Autodesk Inventor part; units mm, degrees
(part 3 of 3)
  spline S71 degree 3 poles (611.9865, 25.0748) (610.6815, 25.5594) (608.0715, 26.5286) (604.1238, 27.8919) (600.1524, 29.1842) (596.1558, 30.3968) (592.133, 31.5183) (589.1016, 32.3079) (587.0663, 32.7741) (586.2405, 33.0576) (585.6183, 33.3719) (585.1825, 33.6602) (584.7659, 33.9763) (584.3992, 34.3495) (584.0638, 34.7502) (583.7778, 35.1888) (583.5529, 35.6608) (583.3681, 36.1496) (583.2424, 36.658) (583.1703, 37.3513) (583.1308, 38.2204) (583.0565, 39.0872) (583.0375, 39.784) (583.0958, 40.3045) (583.2151, 40.8133) (583.3766, 41.3106) (583.6029, 41.7827) (583.883, 42.2238) (584.1979, 42.6417) (584.5697, 43.0094) (584.9641, 43.3521) (585.54, 43.745) (586.3218, 44.1338) (588.2787, 44.8617) (591.1811, 46.0402) (595.0232, 47.6772) (598.8274, 49.4011) (602.596, 51.2007) (606.332, 53.0676) (608.7932, 54.3692) (610.0238, 55.02) knots 0 0 0 0 0.062504 0.125008 0.187512 0.250016 0.31252 0.375023 0.390648 0.406259 0.414073 0.421883 0.429693 0.437504 0.445316 0.453129 0.460938 0.468749 0.476563 0.484374 0.5 0.515626 0.523437 0.531251 0.539062 0.546871 0.554684 0.562496 0.570307 0.578117 0.585927 0.593741 0.609352 0.624977 0.68748 0.749984 0.812488 0.874992 0.937496 1 1 1 1 projected
  arc A75 (610.0238, 55.02) -> (609.0362, 65.0469) centre (0, 0) ccw projected
  spline S72 degree 3 poles (609.0362, 65.0469) (607.7023, 65.4451) (605.0345, 66.2416) (601.0061, 67.3437) (596.9587, 68.3736) (592.8914, 69.3221) (588.8038, 70.1781) (585.7272, 70.7678) (583.6659, 71.0999) (582.8232, 71.3287) (582.1818, 71.6018) (581.7281, 71.8609) (581.2917, 72.1491) (580.9014, 72.4975) (580.5405, 72.8754) (580.2265, 73.2943) (579.9711, 73.7506) (579.7548, 74.2263) (579.5961, 74.7254) (579.4788, 75.4125) (579.3825, 76.2772) (579.2517, 77.1372) (579.1872, 77.8313) (579.2113, 78.3545) (579.2971, 78.87) (579.4257, 79.3768) (579.6206, 79.8627) (579.8713, 80.3212) (580.1582, 80.7587) (580.5051, 81.15) (580.8763, 81.5177) (581.4252, 81.9475) (582.1799, 82.3866) (584.0851, 83.2409) (586.9042, 84.6067) (590.631, 86.4915) (594.3142, 88.4605) (597.9571, 90.5028) (601.5631, 92.61) (603.9338, 94.0698) (605.1192, 94.7997) knots 0 0 0 0 0.062504 0.125008 0.187512 0.250016 0.31252 0.375023 0.390648 0.406259 0.414073 0.421883 0.429693 0.437504 0.445316 0.453129 0.460938 0.468749 0.476563 0.484374 0.5 0.515626 0.523437 0.531251 0.539062 0.546871 0.554684 0.562496 0.570307 0.578117 0.585927 0.593741 0.609352 0.624977 0.68748 0.749984 0.812488 0.874992 0.937496 1 1 1 1 projected
  arc A76 (605.1192, 94.7997) -> (603.478, 104.7405) centre (0, 0) ccw projected
  spline S73 degree 3 poles (603.478, 104.7405) (602.1209, 105.0506) (599.4067, 105.6709) (595.3148, 106.5072) (591.2087, 107.2701) (587.088, 107.9507) (582.9532, 108.5375) (579.8447, 108.9247) (577.766, 109.1212) (576.9102, 109.2945) (576.2523, 109.525) (575.7826, 109.7539) (575.3283, 110.0129) (574.916, 110.335) (574.5313, 110.6885) (574.1905, 111.086) (573.9058, 111.5246) (573.6589, 111.9851) (573.4678, 112.4728) (573.3059, 113.1508) (573.1532, 114.0073) (572.9665, 114.857) (572.8567, 115.5453) (572.8465, 116.069) (572.8985, 116.5889) (572.9936, 117.1031) (573.1564, 117.6007) (573.3765, 118.0746) (573.6342, 118.53) (573.9548, 118.9431) (574.3011, 119.3343) (574.8207, 119.7991) (575.5451, 120.2866) (577.3903, 121.2637) (580.114, 122.811) (583.7096, 124.9355) (587.2562, 127.1411) (590.7577, 129.4173) (594.2181, 131.7558) (596.4883, 133.3675) (597.6234, 134.1734) knots 0 0 0 0 0.062504 0.125008 0.187512 0.250016 0.31252 0.375023 0.390648 0.406259 0.414073 0.421883 0.429693 0.437504 0.445316 0.453129 0.460938 0.468749 0.476563 0.484374 0.5 0.515626 0.523437 0.531251 0.539062 0.546871 0.554684 0.562496 0.570307 0.578117 0.585927 0.593741 0.609352 0.624977 0.68748 0.749984 0.812488 0.874992 0.937496 1 1 1 1 projected
  arc A77 (597.6234, 134.1734) -> (595.3355, 143.9856) centre (0, 0) ccw projected
  spline S74 degree 3 poles (595.3355, 143.9856) (593.9611, 144.2063) (591.2121, 144.6477) (587.0743, 145.2146) (582.9271, 145.7074) (578.7707, 146.1169) (574.6064, 146.4321) (571.4792, 146.6151) (569.3921, 146.6753) (568.5268, 146.7922) (567.8552, 146.9792) (567.3716, 147.1769) (566.9013, 147.4056) (566.4688, 147.7001) (566.0618, 148.0277) (565.6957, 148.402) (565.383, 148.8211) (565.1064, 149.2645) (564.8839, 149.7386) (564.6779, 150.4045) (564.4696, 151.2492) (564.2277, 152.0848) (564.0731, 152.7645) (564.0288, 153.2864) (564.0466, 153.8087) (564.1079, 154.3279) (564.2377, 154.8352) (564.4264, 155.3224) (564.6538, 155.7937) (564.9466, 156.2269) (565.2666, 156.6399) (565.7548, 157.1376) (566.4457, 157.6715) (568.223, 158.7672) (570.8398, 160.4893) (574.2886, 162.8444) (577.6834, 165.2773) (581.0285, 167.7776) (584.3286, 170.3374) (586.4885, 172.0942) (587.5685, 172.9726) knots 0 0 0 0 0.062504 0.125008 0.187512 0.250016 0.31252 0.375023 0.390648 0.406259 0.414073 0.421883 0.429693 0.437504 0.445316 0.453129 0.460938 0.468749 0.476563 0.484374 0.5 0.515626 0.523437 0.531251 0.539062 0.546871 0.554684 0.562496 0.570307 0.578117 0.585927 0.593741 0.609352 0.624977 0.68748 0.749984 0.812488 0.874992 0.937496 1 1 1 1 projected
  arc A78 (587.5685, 172.9726) -> (584.6438, 182.6141) centre (0, 0) ccw projected
  spline S75 degree 3 poles (584.6438, 182.6141) (583.2578, 182.7445) (580.4859, 183.0051) (576.3198, 183.3002) (572.1493, 183.5207) (567.975, 183.6575) (563.799, 183.6996) (560.6665, 183.6777) (558.58, 183.6013) (557.7089, 183.6613) (557.0265, 183.804) (556.531, 183.9696) (556.0468, 184.1671) (555.5959, 184.4327) (555.1683, 184.733) (554.7786, 185.0826) (554.4391, 185.4802) (554.1341, 185.9046) (553.8811, 186.3632) (553.632, 187.0142) (553.3689, 187.8434) (553.0728, 188.6615) (552.8741, 189.3296) (552.7957, 189.8475) (552.7793, 190.3698) (552.8066, 190.8919) (552.903, 191.4066) (553.0594, 191.9051) (553.2554, 192.3902) (553.5193, 192.8417) (553.8116, 193.2747) (554.2662, 193.8033) (554.9207, 194.3813) (556.6226, 195.5908) (559.121, 197.4804) (562.4085, 200.056) (565.6369, 202.7057) (568.8113, 205.4194) (571.9369, 208.1897) (573.9773, 210.0839) (574.9975, 211.031) knots 0 0 0 0 0.062504 0.125008 0.187512 0.250016 0.31252 0.375023 0.390648 0.406259 0.414073 0.421883 0.429693 0.437504 0.445316 0.453129 0.460938 0.468749 0.476563 0.484374 0.5 0.515626 0.523437 0.531251 0.539062 0.546871 0.554684 0.562496 0.570307 0.578117 0.585927 0.593741 0.609352 0.624977 0.68748 0.749984 0.812488 0.874992 0.937496 1 1 1 1 projected
  arc A79 (574.9975, 211.031) -> (571.4485, 220.4607) centre (0, 0) ccw projected
  spline S76 degree 3 poles (571.4485, 220.4607) (570.0569, 220.5001) (567.2739, 220.5789) (563.0974, 220.6009) (558.9215, 220.5481) (554.7472, 220.4116) (550.5773, 220.1805) (547.453, 219.9538) (545.3759, 219.741) (544.5028, 219.744) (543.8125, 219.8417) (543.3072, 219.9746) (542.8111, 220.14) (542.3439, 220.3755) (541.8976, 220.6472) (541.4858, 220.9705) (541.121, 221.3452) (540.7889, 221.7487) (540.5064, 222.1897) (540.2153, 222.823) (539.8985, 223.6333) (539.5496, 224.4302) (539.3076, 225.0839) (539.1955, 225.5955) (539.145, 226.1157) (539.138, 226.6385) (539.2006, 227.1583) (539.3241, 227.666) (539.4879, 228.1629) (539.7217, 228.6307) (539.9851, 229.0819) (540.4041, 229.6391) (541.0194, 230.2586) (542.6385, 231.5769) (545.0081, 233.6258) (548.12, 236.411) (551.1682, 239.2661) (554.1584, 242.1816) (557.0961, 245.1504) (559.0082, 247.174) (559.9643, 248.1858) knots 0 0 0 0 0.062504 0.125008 0.187512 0.250016 0.31252 0.375023 0.390648 0.406259 0.414073 0.421883 0.429693 0.437504 0.445316 0.453129 0.460938 0.468749 0.476563 0.484374 0.5 0.515626 0.523437 0.531251 0.539062 0.546871 0.554684 0.562496 0.570307 0.578117 0.585927 0.593741 0.609352 0.624977 0.68748 0.749984 0.812488 0.874992 0.937496 1 1 1 1 projected
  arc A80 (559.9643, 248.1858) -> (555.8061, 257.3632) centre (0, 0) ccw projected
  spline S77 degree 3 poles (555.8061, 257.3632) (554.415, 257.3115) (551.6328, 257.2081) (547.4638, 256.9569) (543.3002, 256.6311) (539.1438, 256.2219) (534.998, 255.7186) (531.8952, 255.288) (529.8365, 254.9399) (528.965, 254.8857) (528.2698, 254.9381) (527.7569, 255.0376) (527.2511, 255.1702) (526.7694, 255.3746) (526.3063, 255.6166) (525.8742, 255.9123) (525.4858, 256.2623) (525.128, 256.6432) (524.8173, 257.0648) (524.4854, 257.6777) (524.1162, 258.4655) (523.7159, 259.2379) (523.4317, 259.8744) (523.2864, 260.3776) (523.202, 260.8933) (523.1608, 261.4146) (523.1892, 261.9374) (523.2793, 262.4521) (523.4103, 262.9586) (523.613, 263.4407) (523.8463, 263.9082) (524.2279, 264.4916) (524.8014, 265.15) (526.3309, 266.5713) (528.5613, 268.7708) (531.4845, 271.7535) (534.3394, 274.802) (537.1325, 277.9068) (539.8697, 281.0613) (541.6454, 283.2057) (542.5333, 284.2779) knots 0 0 0 0 0.062504 0.125008 0.187512 0.250016 0.31252 0.375023 0.390648 0.406259 0.414073 0.421883 0.429693 0.437504 0.445316 0.453129 0.460938 0.468749 0.476563 0.484374 0.5 0.515626 0.523437 0.531251 0.539062 0.546871 0.554684 0.562496 0.570307 0.578117 0.585927 0.593741 0.609352 0.624977 0.68748 0.749984 0.812488 0.874992 0.937496 1 1 1 1 projected
  arc A81 (542.5333, 284.2779) -> (537.7837, 293.1636) centre (0, 0) ccw projected
  spline S78 degree 3 poles (537.7837, 293.1636) (536.399, 293.021) (533.6295, 292.7359) (529.4859, 292.2126) (525.3525, 291.6152) (521.2318, 290.935) (517.1277, 290.1616) (514.0597, 289.529) (512.0282, 289.047) (511.1621, 288.936) (510.465, 288.9427) (509.9467, 289.0085) (509.4333, 289.1077) (508.9393, 289.2802) (508.4613, 289.4913) (508.0108, 289.7582) (507.6003, 290.082) (507.2184, 290.4387) (506.8808, 290.8391) (506.5095, 291.429) (506.0896, 292.191) (505.6397, 292.9356) (505.3144, 293.5521) (505.1365, 294.0447) (505.0185, 294.5538) (504.9434, 295.0712) (504.9375, 295.5947) (504.9937, 296.1142) (505.0913, 296.6283) (505.2621, 297.1225) (505.4643, 297.6043) (505.8069, 298.2114) (506.3361, 298.9059) (507.7693, 300.4243) (509.8512, 302.765) (512.573, 305.9324) (515.2224, 309.161) (517.8064, 312.4419) (520.3315, 315.7687) (521.9632, 318.0246) (522.779, 319.1526) knots 0 0 0 0 0.062504 0.125008 0.187512 0.250016 0.31252 0.375023 0.390648 0.406259 0.414073 0.421883 0.429693 0.437504 0.445316 0.453129 0.460938 0.468749 0.476563 0.484374 0.5 0.515626 0.523437 0.531251 0.539062 0.546871 0.554684 0.562496 0.570307 0.578117 0.585927 0.593741 0.609352 0.624977 0.68748 0.749984 0.812488 0.874992 0.937496 1 1 1 1 projected
  arc A82 (522.779, 319.1526) -> (517.4585, 327.7086) centre (0, 0) ccw projected
  spline S79 degree 3 poles (517.4585, 327.7086) (516.086, 327.4758) (513.3411, 327.0102) (509.2406, 326.217) (505.1551, 325.3505) (501.0877, 324.4023) (497.043, 323.3621) (494.023, 322.5302) (492.0273, 321.9163) (491.1704, 321.7489) (490.4743, 321.7101) (489.9528, 321.7418) (489.434, 321.8073) (488.9298, 321.9471) (488.439, 322.1265) (487.9721, 322.3633) (487.5412, 322.6596) (487.1368, 322.9905) (486.7737, 323.368) (486.3646, 323.9323) (485.8958, 324.6652) (485.3981, 325.3788) (485.0333, 325.9727) (484.8235, 326.4526) (484.6725, 326.9529) (484.5637, 327.4643) (484.5236, 327.9863) (484.5457, 328.5084) (484.6094, 329.0277) (484.7475, 329.5321) (484.9178, 330.0261) (485.22, 330.6543) (485.7026, 331.3819) (487.0335, 332.9907) (488.9578, 335.4626) (491.4666, 338.8013) (493.8992, 342.1963) (496.2631, 345.6391) (498.5651, 349.1239) (500.0458, 351.4817) (500.7861, 352.6606) knots 0 0 0 0 0.062504 0.125008 0.187512 0.250016 0.31252 0.375023 0.390648 0.406259 0.414073 0.421883 0.429693 0.437504 0.445316 0.453129 0.460938 0.468749 0.476563 0.484374 0.5 0.515626 0.523437 0.531251 0.539062 0.546871 0.554684 0.562496 0.570307 0.578117 0.585927 0.593741 0.609352 0.624977 0.68748 0.749984 0.812488 0.874992 0.937496 1 1 1 1 projected
  arc A83 (500.7861, 352.6606) -> (494.9174, 360.8504) centre (0, 0) ccw projected
  spline S80 degree 3 poles (494.9174, 360.8504) (493.5631, 360.5283) (490.8545, 359.8842) (486.8147, 358.8244) (482.7946, 357.6926) (478.7979, 356.4804) (474.8299, 355.1779) (471.8707, 354.1503) (469.9195, 353.4072) (469.0753, 353.1841) (468.3833, 353.0998) (467.8609, 353.0974) (467.3389, 353.1288) (466.8266, 353.2353) (466.3252, 353.3822) (465.8437, 353.588) (465.3944, 353.8554) (464.9692, 354.1592) (464.5822, 354.5121) (464.1371, 355.0485) (463.6214, 355.7492) (463.0781, 356.4287) (462.6752, 356.9975) (462.4345, 357.4626) (462.251, 357.952) (462.109, 358.4552) (462.0348, 358.9735) (462.0227, 359.4958) (462.0524, 360.0182) (462.1572, 360.5306) (462.2948, 361.0346) (462.5553, 361.6812) (462.9893, 362.4389) (464.2121, 364.1313) (465.9706, 366.7237) (468.2556, 370.2193) (470.461, 373.7661) (472.5947, 377.3563) (474.6639, 380.9841) (475.9871, 383.4337) (476.6488, 384.6585) knots 0 0 0 0 0.062504 0.125008 0.187512 0.250016 0.31252 0.375023 0.390648 0.406259 0.414073 0.421883 0.429693 0.437504 0.445316 0.453129 0.460938 0.468749 0.476563 0.484374 0.5 0.515626 0.523437 0.531251 0.539062 0.546871 0.554684 0.562496 0.570307 0.578117 0.585927 0.593741 0.609352 0.624977 0.68748 0.749984 0.812488 0.874992 0.937496 1 1 1 1 projected
  arc A84 (476.6488, 384.6585) -> (470.257, 392.4469) centre (0, 0) ccw projected
  spline S81 degree 3 poles (470.257, 392.4469) (468.9267, 392.037) (466.266, 391.217) (462.3041, 389.8954) (458.3667, 388.503) (454.4578, 387.032) (450.5835, 385.4728) (447.6979, 384.2539) (445.7994, 383.3848) (444.9717, 383.1069) (444.2867, 382.9776) (443.7655, 382.941) (443.2425, 382.9381) (442.7244, 383.0109) (442.2144, 383.1247) (441.7205, 383.2986) (441.2547, 383.5361) (440.8106, 383.8114) (440.4013, 384.1382) (439.922, 384.6444) (439.3616, 385.3098) (438.775, 385.9523) (438.3358, 386.4935) (438.0652, 386.9419) (437.8501, 387.4182) (437.6755, 387.9111) (437.5676, 388.4234) (437.5214, 388.9439) (437.5168, 389.4671) (437.5879, 389.9852) (437.6922, 390.4971) (437.9098, 391.1594) (438.2934, 391.9438) (439.4028, 393.7126) (440.988, 396.4144) (443.0396, 400.0521) (445.0082, 403.7355) (446.9025, 407.4575) (448.73, 411.2129) (449.8903, 413.7438) (450.4704, 415.0093) knots 0 0 0 0 0.062504 0.125008 0.187512 0.250016 0.31252 0.375023 0.390648 0.406259 0.414073 0.421883 0.429693 0.437504 0.445316 0.453129 0.460938 0.468749 0.476563 0.484374 0.5 0.515626 0.523437 0.531251 0.539062 0.546871 0.554684 0.562496 0.570307 0.578117 0.585927 0.593741 0.609352 0.624977 0.68748 0.749984 0.812488 0.874992 0.937496 1 1 1 1 projected
  arc A85 (450.4704, 415.0093) -> (443.5829, 422.363) centre (0, 0) ccw projected
  spline S82 degree 3 poles (443.5829, 422.363) (442.2822, 421.8669) (439.6808, 420.8747) (435.8139, 419.2967) (431.976, 417.6498) (428.1717, 415.9263) (424.4077, 414.1171) (421.6079, 412.712) (419.7704, 411.7206) (418.9626, 411.3892) (418.2875, 411.2153) (417.7698, 411.1447) (417.2482, 411.1077) (416.7264, 411.1464) (416.21, 411.2266) (415.7059, 411.3678) (415.2255, 411.5743) (414.7643, 411.82) (414.3345, 412.1194) (413.8232, 412.5931) (413.2204, 413.2204) (412.5931, 413.8232) (412.1194, 414.3345) (411.82, 414.7643) (411.5743, 415.2255) (411.3678, 415.7059) (411.2266, 416.21) (411.1464, 416.7264) (411.1077, 417.2482) (411.1447, 417.7698) (411.2153, 418.2875) (411.3892, 418.9626) (411.7206, 419.7704) (412.712, 421.6079) (414.1171, 424.4077) (415.9263, 428.1717) (417.6498, 431.976) (419.2967, 435.8139) (420.8747, 439.6808) (421.8669, 442.2822) (422.363, 443.5829) knots 0 0 0 0 0.062504 0.125008 0.187512 0.250016 0.31252 0.375023 0.390648 0.406259 0.414073 0.421883 0.429693 0.437504 0.445316 0.453129 0.460938 0.468749 0.476563 0.484374 0.5 0.515626 0.523437 0.531251 0.539062 0.546871 0.554684 0.562496 0.570307 0.578117 0.585927 0.593741 0.609352 0.624977 0.68748 0.749984 0.812488 0.874992 0.937496 1 1 1 1 projected
  arc A86 (422.363, 443.5829) -> (415.0093, 450.4704) centre (0, 0) ccw projected
  spline S83 degree 3 poles (415.0093, 450.4704) (413.7438, 449.8903) (411.2129, 448.73) (407.4575, 446.9025) (403.7355, 445.0082) (400.0521, 443.0396) (396.4144, 440.988) (393.7126, 439.4028) (391.9438, 438.2934) (391.1594, 437.9098) (390.4971, 437.6922) (389.9852, 437.5879) (389.4671, 437.5168) (388.9439, 437.5214) (388.4234, 437.5676) (387.9111, 437.6755) (387.4182, 437.8501) (386.9419, 438.0652) (386.4935, 438.3358) (385.9523, 438.775) (385.3098, 439.3616) (384.6444, 439.922) (384.1382, 440.4013) (383.8114, 440.8106) (383.5361, 441.2547) (383.2986, 441.7205) (383.1247, 442.2144) (383.0109, 442.7244) (382.9381, 443.2425) (382.941, 443.7655) (382.9776, 444.2867) (383.1069, 444.9717) (383.3848, 445.7994) (384.2539, 447.6979) (385.4728, 450.5835) (387.032, 454.4578) (388.503, 458.3667) (389.8954, 462.3041) (391.217, 466.266) (392.037, 468.9267) (392.4469, 470.257) knots 0 0 0 0 0.062504 0.125008 0.187512 0.250016 0.31252 0.375023 0.390648 0.406259 0.414073 0.421883 0.429693 0.437504 0.445316 0.453129 0.460938 0.468749 0.476563 0.484374 0.5 0.515626 0.523437 0.531251 0.539062 0.546871 0.554684 0.562496 0.570307 0.578117 0.585927 0.593741 0.609352 0.624977 0.68748 0.749984 0.812488 0.874992 0.937496 1 1 1 1 projected
  arc A87 (392.4469, 470.257) -> (384.6585, 476.6488) centre (0, 0) ccw projected
  spline S84 degree 3 poles (384.6585, 476.6488) (383.4337, 475.9871) (380.9841, 474.6639) (377.3563, 472.5947) (373.7661, 470.461) (370.2193, 468.2556) (366.7237, 465.9706) (364.1313, 464.2121) (362.4389, 462.9893) (361.6812, 462.5553) (361.0346, 462.2948) (360.5306, 462.1572) (360.0182, 462.0524) (359.4958, 462.0227) (358.9735, 462.0348) (358.4552, 462.109) (357.952, 462.251) (357.4626, 462.4345) (356.9975, 462.6752) (356.4287, 463.0781) (355.7492, 463.6214) (355.0485, 464.1371) (354.5121, 464.5822) (354.1592, 464.9692) (353.8554, 465.3944) (353.588, 465.8437) (353.3822, 466.3252) (353.2353, 466.8266) (353.1288, 467.3389) (353.0974, 467.8609) (353.0998, 468.3833) (353.1841, 469.0753) (353.4072, 469.9195) (354.1503, 471.8707) (355.1779, 474.8299) (356.4804, 478.7979) (357.6926, 482.7946) (358.8244, 486.8147) (359.8842, 490.8545) (360.5283, 493.5631) (360.8504, 494.9174) knots 0 0 0 0 0.062504 0.125008 0.187512 0.250016 0.31252 0.375023 0.390648 0.406259 0.414073 0.421883 0.429693 0.437504 0.445316 0.453129 0.460938 0.468749 0.476563 0.484374 0.5 0.515626 0.523437 0.531251 0.539062 0.546871 0.554684 0.562496 0.570307 0.578117 0.585927 0.593741 0.609352 0.624977 0.68748 0.749984 0.812488 0.874992 0.937496 1 1 1 1 projected
  arc A88 (360.8504, 494.9174) -> (352.6606, 500.7861) centre (0, 0) ccw projected
  spline S85 degree 3 poles (352.6606, 500.7861) (351.4817, 500.0458) (349.1239, 498.5651) (345.6391, 496.2631) (342.1963, 493.8992) (338.8013, 491.4666) (335.4626, 488.9578) (332.9907, 487.0335) (331.3819, 485.7026) (330.6543, 485.22) (330.0261, 484.9178) (329.5321, 484.7475) (329.0277, 484.6094) (328.5084, 484.5457) (327.9863, 484.5236) (327.4643, 484.5637) (326.9529, 484.6725) (326.4526, 484.8235) (325.9727, 485.0333) (325.3788, 485.3981) (324.6652, 485.8958) (323.9323, 486.3646) (323.368, 486.7737) (322.9905, 487.1368) (322.6596, 487.5412) (322.3633, 487.9721) (322.1265, 488.439) (321.9471, 488.9298) (321.8073, 489.434) (321.7418, 489.9528) (321.7101, 490.4743) (321.7489, 491.1704) (321.9163, 492.0273) (322.5302, 494.023) (323.3621, 497.043) (324.4023, 501.0877) (325.3505, 505.1551) (326.217, 509.2406) (327.0102, 513.3411) (327.4758, 516.086) (327.7086, 517.4585) knots 0 0 0 0 0.062504 0.125008 0.187512 0.250016 0.31252 0.375023 0.390648 0.406259 0.414073 0.421883 0.429693 0.437504 0.445316 0.453129 0.460938 0.468749 0.476563 0.484374 0.5 0.515626 0.523437 0.531251 0.539062 0.546871 0.554684 0.562496 0.570307 0.578117 0.585927 0.593741 0.609352 0.624977 0.68748 0.749984 0.812488 0.874992 0.937496 1 1 1 1 projected
  arc A89 (327.7086, 517.4585) -> (319.1526, 522.779) centre (0, 0) ccw projected
  spline S86 degree 3 poles (319.1526, 522.779) (318.0246, 521.9632) (315.7687, 520.3315) (312.4419, 517.8064) (309.161, 515.2224) (305.9324, 512.573) (302.765, 509.8512) (300.4243, 507.7693) (298.9059, 506.3361) (298.2114, 505.8069) (297.6043, 505.4643) (297.1225, 505.2621) (296.6283, 505.0913) (296.1142, 504.9937) (295.5947, 504.9375) (295.0712, 504.9434) (294.5538, 505.0185) (294.0447, 505.1365) (293.5521, 505.3144) (292.9356, 505.6397) (292.191, 506.0896) (291.429, 506.5095) (290.8391, 506.8808) (290.4387, 507.2184) (290.082, 507.6003) (289.7582, 508.0108) (289.4913, 508.4613) (289.2802, 508.9393) (289.1077, 509.4333) (289.0085, 509.9467) (288.9427, 510.465) (288.936, 511.1621) (289.047, 512.0282) (289.529, 514.0597) (290.1616, 517.1277) (290.935, 521.2318) (291.6152, 525.3525) (292.2126, 529.4859) (292.7359, 533.6295) (293.021, 536.399) (293.1636, 537.7837) knots 0 0 0 0 0.062504 0.125008 0.187512 0.250016 0.31252 0.375023 0.390648 0.406259 0.414073 0.421883 0.429693 0.437504 0.445316 0.453129 0.460938 0.468749 0.476563 0.484374 0.5 0.515626 0.523437 0.531251 0.539062 0.546871 0.554684 0.562496 0.570307 0.578117 0.585927 0.593741 0.609352 0.624977 0.68748 0.749984 0.812488 0.874992 0.937496 1 1 1 1 projected
  arc A90 (293.1636, 537.7837) -> (284.2779, 542.5333) centre (0, 0) ccw projected
  spline S87 degree 3 poles (284.2779, 542.5333) (283.2057, 541.6454) (281.0613, 539.8697) (277.9068, 537.1325) (274.802, 534.3394) (271.7535, 531.4845) (268.7708, 528.5613) (266.5713, 526.3309) (265.15, 524.8014) (264.4916, 524.2279) (263.9082, 523.8463) (263.4407, 523.613) (262.9586, 523.4103) (262.4521, 523.2793) (261.9374, 523.1892) (261.4146, 523.1608) (260.8933, 523.202) (260.3776, 523.2864) (259.8744, 523.4317) (259.2379, 523.7159) (258.4655, 524.1162) (257.6777, 524.4854) (257.0648, 524.8173) (256.6432, 525.128) (256.2623, 525.4858) (255.9123, 525.8742) (255.6166, 526.3063) (255.3746, 526.7694) (255.1702, 527.2511) (255.0376, 527.7569) (254.9381, 528.2698) (254.8857, 528.965) (254.9399, 529.8365) (255.288, 531.8952) (255.7186, 534.998) (256.2219, 539.1438) (256.6311, 543.3002) (256.9569, 547.4638) (257.2081, 551.6328) (257.3115, 554.415) (257.3632, 555.8061) knots 0 0 0 0 0.062504 0.125008 0.187512 0.250016 0.31252 0.375023 0.390648 0.406259 0.414073 0.421883 0.429693 0.437504 0.445316 0.453129 0.460938 0.468749 0.476563 0.484374 0.5 0.515626 0.523437 0.531251 0.539062 0.546871 0.554684 0.562496 0.570307 0.578117 0.585927 0.593741 0.609352 0.624977 0.68748 0.749984 0.812488 0.874992 0.937496 1 1 1 1 projected
  arc A91 (257.3632, 555.8061) -> (248.1858, 559.9643) centre (0, 0) ccw projected
  spline S88 degree 3 poles (248.1858, 559.9643) (247.174, 559.0082) (245.1504, 557.0961) (242.1816, 554.1584) (239.2661, 551.1682) (236.411, 548.12) (233.6258, 545.0081) (231.5769, 542.6385) (230.2586, 541.0194) (229.6391, 540.4041) (229.0819, 539.9851) (228.6307, 539.7217) (228.1629, 539.4879) (227.666, 539.3241) (227.1583, 539.2006) (226.6385, 539.138) (226.1157, 539.145) (225.5955, 539.1955) (225.0839, 539.3076) (224.4302, 539.5496) (223.6333, 539.8985) (222.823, 540.2153) (222.1897, 540.5064) (221.7487, 540.7889) (221.3452, 541.121) (220.9705, 541.4858) (220.6472, 541.8976) (220.3755, 542.3439) (220.14, 542.8111) (219.9746, 543.3072) (219.8417, 543.8125) (219.744, 544.5028) (219.741, 545.3759) (219.9538, 547.453) (220.1805, 550.5773) (220.4116, 554.7472) (220.5481, 558.9215) (220.6009, 563.0974) (220.5789, 567.2739) (220.5001, 570.0569) (220.4607, 571.4485) knots 0 0 0 0 0.062504 0.125008 0.187512 0.250016 0.31252 0.375023 0.390648 0.406259 0.414073 0.421883 0.429693 0.437504 0.445316 0.453129 0.460938 0.468749 0.476563 0.484374 0.5 0.515626 0.523437 0.531251 0.539062 0.546871 0.554684 0.562496 0.570307 0.578117 0.585927 0.593741 0.609352 0.624977 0.68748 0.749984 0.812488 0.874992 0.937496 1 1 1 1 projected
  arc A92 (220.4607, 571.4485) -> (211.031, 574.9975) centre (0, 0) ccw projected
  spline S89 degree 3 poles (211.031, 574.9975) (210.0839, 573.9773) (208.1897, 571.9369) (205.4194, 568.8113) (202.7057, 565.6369) (200.056, 562.4085) (197.4804, 559.121) (195.5908, 556.6226) (194.3813, 554.9207) (193.8033, 554.2662) (193.2747, 553.8116) (192.8417, 553.5193) (192.3902, 553.2554) (191.9051, 553.0594) (191.4066, 552.903) (190.8919, 552.8066) (190.3698, 552.7793) (189.8475, 552.7957) (189.3296, 552.8741) (188.6615, 553.0728) (187.8434, 553.3689) (187.0142, 553.632) (186.3632, 553.8811) (185.9046, 554.1341) (185.4802, 554.4391) (185.0826, 554.7786) (184.733, 555.1683) (184.4327, 555.5959) (184.1671, 556.0468) (183.9696, 556.531) (183.804, 557.0265) (183.6613, 557.7089) (183.6013, 558.58) (183.6777, 560.6665) (183.6996, 563.799) (183.6575, 567.975) (183.5207, 572.1493) (183.3002, 576.3198) (183.0051, 580.4859) (182.7445, 583.2578) (182.6141, 584.6438) knots 0 0 0 0 0.062504 0.125008 0.187512 0.250016 0.31252 0.375023 0.390648 0.406259 0.414073 0.421883 0.429693 0.437504 0.445316 0.453129 0.460938 0.468749 0.476563 0.484374 0.5 0.515626 0.523437 0.531251 0.539062 0.546871 0.554684 0.562496 0.570307 0.578117 0.585927 0.593741 0.609352 0.624977 0.68748 0.749984 0.812488 0.874992 0.937496 1 1 1 1 projected
  arc A93 (182.6141, 584.6438) -> (172.9726, 587.5685) centre (0, 0) ccw projected
  spline S90 degree 3 poles (172.9726, 587.5685) (172.0942, 586.4885) (170.3374, 584.3286) (167.7776, 581.0285) (165.2773, 577.6834) (162.8444, 574.2886) (160.4893, 570.8398) (158.7672, 568.223) (157.6715, 566.4457) (157.1376, 565.7548) (156.6399, 565.2666) (156.2269, 564.9466) (155.7937, 564.6538) (155.3224, 564.4264) (154.8352, 564.2377) (154.3279, 564.1079) (153.8087, 564.0466) (153.2864, 564.0288) (152.7645, 564.0731) (152.0848, 564.2277) (151.2492, 564.4696) (150.4045, 564.6779) (149.7386, 564.8839) (149.2645, 565.1064) (148.8211, 565.383) (148.402, 565.6957) (148.0277, 566.0618) (147.7001, 566.4688) (147.4056, 566.9013) (147.1769, 567.3716) (146.9792, 567.8552) (146.7922, 568.5268) (146.6753, 569.3921) (146.6151, 571.4792) (146.4321, 574.6064) (146.1169, 578.7707) (145.7074, 582.9271) (145.2146, 587.0743) (144.6477, 591.2121) (144.2063, 593.9611) (143.9856, 595.3355) knots 0 0 0 0 0.062504 0.125008 0.187512 0.250016 0.31252 0.375023 0.390648 0.406259 0.414073 0.421883 0.429693 0.437504 0.445316 0.453129 0.460938 0.468749 0.476563 0.484374 0.5 0.515626 0.523437 0.531251 0.539062 0.546871 0.554684 0.562496 0.570307 0.578117 0.585927 0.593741 0.609352 0.624977 0.68748 0.749984 0.812488 0.874992 0.937496 1 1 1 1 projected
  arc A94 (143.9856, 595.3355) -> (134.1734, 597.6234) centre (0, 0) ccw projected
  spline S91 degree 3 poles (134.1734, 597.6234) (133.3675, 596.4883) (131.7558, 594.2181) (129.4173, 590.7577) (127.1411, 587.2562) (124.9355, 583.7096) (122.811, 580.114) (121.2637, 577.3903) (120.2866, 575.5451) (119.7991, 574.8207) (119.3343, 574.3011) (118.9431, 573.9548) (118.53, 573.6342) (118.0746, 573.3765) (117.6007, 573.1564) (117.1031, 572.9936) (116.5889, 572.8985) (116.069, 572.8465) (115.5453, 572.8567) (114.857, 572.9665) (114.0073, 573.1532) (113.1508, 573.3059) (112.4728, 573.4678) (111.9851, 573.6589) (111.5246, 573.9058) (111.086, 574.1905) (110.6885, 574.5313) (110.335, 574.916) (110.0129, 575.3283) (109.7539, 575.7826) (109.525, 576.2523) (109.2945, 576.9102) (109.1212, 577.766) (108.9247, 579.8447) (108.5375, 582.9532) (107.9507, 587.088) (107.2701, 591.2087) (106.5072, 595.3148) (105.6709, 599.4067) (105.0506, 602.1209) (104.7405, 603.478) knots 0 0 0 0 0.062504 0.125008 0.187512 0.250016 0.31252 0.375023 0.390648 0.406259 0.414073 0.421883 0.429693 0.437504 0.445316 0.453129 0.460938 0.468749 0.476563 0.484374 0.5 0.515626 0.523437 0.531251 0.539062 0.546871 0.554684 0.562496 0.570307 0.578117 0.585927 0.593741 0.609352 0.624977 0.68748 0.749984 0.812488 0.874992 0.937496 1 1 1 1 projected
  arc A95 (104.7405, 603.478) -> (94.7997, 605.1192) centre (0, 0) ccw projected
  spline S92 degree 3 poles (94.7997, 605.1192) (94.0698, 603.9338) (92.61, 601.5631) (90.5028, 597.9571) (88.4605, 594.3142) (86.4915, 590.631) (84.6067, 586.9042) (83.2409, 584.0851) (82.3866, 582.1799) (81.9475, 581.4252) (81.5177, 580.8763) (81.15, 580.5051) (80.7587, 580.1582) (80.3212, 579.8713) (79.8627, 579.6206) (79.3768, 579.4257) (78.87, 579.2971) (78.3545, 579.2113) (77.8313, 579.1872) (77.1372, 579.2517) (76.2772, 579.3825) (75.4125, 579.4788) (74.7254, 579.5961) (74.2263, 579.7548) (73.7506, 579.9711) (73.2943, 580.2265) (72.8754, 580.5405) (72.4975, 580.9014) (72.1491, 581.2917) (71.8609, 581.7281) (71.6018, 582.1818) (71.3287, 582.8232) (71.0999, 583.6659) (70.7678, 585.7272) (70.1781, 588.8038) (69.3221, 592.8914) (68.3736, 596.9587) (67.3437, 601.0061) (66.2416, 605.0345) (65.4451, 607.7023) (65.0469, 609.0362) knots 0 0 0 0 0.062504 0.125008 0.187512 0.250016 0.31252 0.375023 0.390648 0.406259 0.414073 0.421883 0.429693 0.437504 0.445316 0.453129 0.460938 0.468749 0.476563 0.484374 0.5 0.515626 0.523437 0.531251 0.539062 0.546871 0.554684 0.562496 0.570307 0.578117 0.585927 0.593741 0.609352 0.624977 0.68748 0.749984 0.812488 0.874992 0.937496 1 1 1 1 projected
  arc A96 (65.0469, 609.0362) -> (55.02, 610.0238) centre (0, 0) ccw projected
  point P0 (-73.0947, 555.2091)
  point P1 (73.0947, 555.2091)
  dimension "d7" = 1120
  dimension "d8" = 15
  constraints: 6 end point, 2 horizontal alignment, 2 vertical alignment, 1 coincident, 1 vertical, 98 other
  measures "d8" angle of L1 L2
extrude "Extrusion3" cut sketch "Sketch2" against normal through all
sketch "Sketch3" plane through (0, 0, 0) normal (0, 0, 1) x (1, 0, 0)
  circle A0 centre (0, 0) radius 566.75 construction
  line L0 (0, 0) -> (0, 566.75) construction
  line L1 (0, 0) -> (55.5512, 564.0209) construction
  line L2 (0, 0) -> (-55.5512, 564.0209) construction
  dimension "d11" = 1133.5
  dimension "d12" = 11.25
  constraints: 6 end point, 3 coincident, 3 point on circle, 1 centre point, 1 vertical, 1 other
  measures "d11" diameter of A0
  measures "d12" angle of L2 L1
hole "Hole1" at (-55.5512, 564.0209, 0) at (55.5512, 564.0209, 0) direction (0, 0, -1) diameter 8 end through all
equation "\"d7\" = Шстр_диам_внутр"
equation "\"Module\" = 12.5"
equation "\"PressureAngle\" = 20deg"
equation "\"UnitProfileClearance\" = 0.25"
equation "\"UnitRoundRadius\" = 0.35"
equation "\"HeadDiameter\" = 1225"
equation "\"RootDiameter\" = 1168.75"
equation "\"BaseDiameter\" = 1127.63114"
equation "\"HelixAngle\" = 0"
equation "\"UnitCorrection\" = 0"
equation "\"UnitAddendumModification\" = 0"
equation "\"CircularPitch\" = 39.269908"
equation "\"UnitBacklashShift\" = 0"
equation "\"TotalToolShift\" = 0"
equation "\"IsInternal\" = 0"
equation "\"Шстр_диам_внутр\" = 1120"
body "Solid1"
